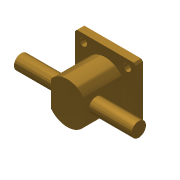
# Autodesk Inventor part: coaxToWaveguidWG18
Saved by Autodesk Inventor 2015 (Build 190159000, 159)
## iProperties
Created: 2014-03-25
Part Number: coaxToWaveguidWG18
Material: Brass, Soft Yellow
Document SubType Name: Modeling
Designer: jad211
Density: 8.47 g/cm^3
Appearance: Brass - Satin
Author: jad211
Autodesk Inventor part; units mm, degrees
ref_plane "YZ Plane" through (0, 0, 0) normal (1, 0, 0) x (0, 1, 0)
ref_plane "XZ Plane" through (0, 0, 0) normal (0, 1, 0) x (-1, 0, 0)
ref_plane "XY Plane" through (0, 0, 0) normal (0, 0, 1) x (1, 0, 0)
sketch "Sketch3" plane through (0, 0, 0) normal (0, 0, 1) x (1, 0, 0)
  line L0 (-15.7, -16.7) -> (15.7, -16.7)
  line L1 (16.7, -15.7) -> (16.7, 15.7)
  line L2 (15.7, 16.7) -> (-15.7, 16.7)
  line L3 (-16.7, 15.7) -> (-16.7, -15.7)
  line L4 (-16.7, -16.7) -> (16.7, 16.7) construction
  line L5 (16.7, -16.7) -> (-16.7, 16.7) construction
  line L6 (-15.7, 16.7) -> (-16.7, 15.7)
  line L7 (15.7, 16.7) -> (16.7, 15.7)
  line L8 (16.7, -15.7) -> (15.7, -16.7)
  line L9 (-16.7, -15.7) -> (-15.7, -16.7)
  line L10 (-4.9497, -8.8994) -> (4.9497, -8.8994)
  line L11 (4.9497, -8.8994) -> (4.9497, 8.8994)
  line L12 (4.9497, 8.8994) -> (-4.9497, 8.8994)
  line L13 (-4.9497, 8.8994) -> (-4.9497, -8.8994)
  line L14 (-4.9497, -8.8994) -> (4.9497, 8.8994) construction
  line L15 (4.9497, -8.8994) -> (-4.9497, 8.8994) construction
  circle A0 centre (-12.14, 12.625) radius 2.045
  circle A1 centre (12.14, 12.625) radius 2.045
  line L16 (0, -16.7) -> (0, 16.7) construction
  circle A2 centre (-12.14, -12.625) radius 2.045
  circle A3 centre (12.14, -12.625) radius 2.045
  line L17 (12.14, 12.625) -> (-12.14, 12.625) construction
  line L18 (-12.14, 12.625) -> (-12.14, -12.625) construction
  line L19 (-12.14, -12.625) -> (12.14, -12.625) construction
  line L20 (12.14, -12.625) -> (12.14, 12.625) construction
  line L21 (-16.7, 0) -> (16.7, 0) construction
  point P0 (0, 0)
  point P1 (0, 0)
  dimension "d0" = 33.4
  dimension "d1" = 33.4
  dimension "d2" = 1
  dimension "d3" = 1
  dimension "d4" = 1
  dimension "d5" = 1
  dimension "d6" = 1
  dimension "d7" = 1
  dimension "d8" = 1
  dimension "d9" = 1
  dimension "d10" = 9.8994
  dimension "d11" = 17.7988
  dimension "d12" = 4.09
  dimension "d13" = 4.09
  dimension "d17" = 4.09
  dimension "d19" = 24.28
  dimension "d20" = 25.25
  dimension "d21" = 4.09
  dimension "d22" = 12.625
  dimension "d23" = 12.14
  constraints: 45 end point, 10 midpoint, 8 point on line, 6 perpendicular, 4 centre point, 4 parallel, 2 horizontal
  measures "d0" distance of L5.end L4.end
  measures "d1" distance of L4.end L5.start
  measures "d2" distance of L2.end L5.end
  measures "d3" distance of L3.start L5.end
  measures "d4" distance of L2.start L4.end
  measures "d5" distance of L1.end L4.end
  measures "d6" distance of L1.start L5.start
  measures "d7" distance of L0.end L5.start
  measures "d8" distance of L3.end L4.start
  measures "d9" distance of L0.start L4.start
  measures "d10" distance of L12.end L11.end
  measures "d11" distance of L11.end L10.end
  measures "d12" diameter of A0
  measures "d13" diameter of A1
  measures "d17" diameter of A2
  measures "d19" distance of L17.start L17.end
  measures "d20" distance of L18.end L17.end
  measures "d21" diameter of A3
  measures "d22" distance from line of L21.start L17
  measures "d23" distance from line of L16 L17.start
extrude "Extrusion1" add sketch "Sketch3" along normal blind 4.1
sketch "Sketch6" plane through (0, 0, 4.1) normal (0, 0, 1) x (1, 0, 0)
  line L0 (9, 7.1589) -> (9, -7.1589)
  line L1 (-9, -7.1589) -> (-9, 7.1589)
  arc A0 (-9, -7.1589) -> (9, -7.1589) centre (0, 0) ccw
  arc A1 (9, 7.1589) -> (-9, 7.1589) centre (0, 0) ccw
  dimension "d66" = 18
  dimension "d67" = 11.5
  dimension "d68" = 11.5
  dimension "d69" = 9
  constraints: 4 end point, 4 point on circle, 2 centre point, 1 coincident, 1 parallel
  measures "d66" distance between parallel lines of L0 L1
  measures "d67" radius of A1
  measures "d68" radius of A0
  measures "d69" distance from line of point (0, 0) L0
extrude "Extrusion4" add sketch "Sketch6" along normal blind 21
sketch "Sketch7" plane through (9, -7.1589, 4.1) normal (1, 0, 0) x (0, 0, -1)
  circle A0 centre (-14, 7.3314) radius 4
  line L0 (-21, 0) -> (-21, 14.3178) projected
  point P0 (4.1, 7.1589)
  dimension "d58" = 8
  dimension "d59" = 7
  constraints: 1 centre point
  measures "d58" diameter of A0
  measures "d59" distance from line of L0 A0.centre
extrude "Extrusion5" add sketch "Sketch7" along normal blind 23.5
sketch "Sketch8" plane through (-9, -7.1589, 4.1) normal (-1, 0, 0) x (0, 0, 1)
  circle A0 centre (14, 7.3314) radius 4
  line L0 (21, 14.3178) -> (21, 0) projected
  point P0 (-4.1, 7.1589)
  dimension "d62" = 8
  dimension "d63" = 7
  constraints: 1 centre point
  measures "d62" diameter of A0
  measures "d63" distance from line of L0 A0.centre
extrude "Extrusion6" add sketch "Sketch8" along normal blind 23.5
equation "\"d3\" = d2"
equation "\"d5\" = d4"
equation "\"d6\" = d4"
equation "\"d7\" = d6"
equation "\"d8\" = d4"
equation "\"d9\" = d8"
body "Solid1"
